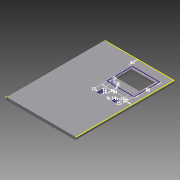
# Autodesk Inventor part: capac frontal
Saved by Autodesk Inventor 2015 SP1 (Build 190203100, 203)
## iProperties
Created: 2015-07-29
Part Number: capac frontal
Material: Generic
Document SubType Name: Modeling
Designer: ubik
Density: 1 g/cm^3
Appearance: Default
Author: ubik
Autodesk Inventor part; units mm, degrees
ref_plane "YZ Plane" through (0, 0, 0) normal (1, 0, 0) x (0, 1, 0)
ref_plane "XZ Plane" through (0, 0, 0) normal (0, 1, 0) x (-1, 0, 0)
ref_plane "XY Plane" through (0, 0, 0) normal (0, 0, 1) x (1, 0, 0)
sketch "Sketch1" plane through (0, 0, 0) normal (0, 0, 1) x (1, 0, 0)
  line L0 (0, 0) -> (240, 0)
  line L1 (240, 0) -> (240, 340)
  line L2 (240, 340) -> (0, 340)
  line L3 (0, 340) -> (0, 0)
  dimension "d0" = 240
  dimension "d1" = 340
  constraints: 8 end point, 2 parallel, 1 horizontal, 1 perpendicular
  measures "d0" distance of L2.end L1.end
  measures "d1" distance of L1.end L0.end
extrude "Extrusion1" add sketch "Sketch1" along normal blind 8
sketch "Sketch2" plane through (0, 0, 8) normal (0, 0, 1) x (1, 0, 0)
  line L0 (126, 310) -> (220, 310)
  line L1 (220, 310) -> (220, 222)
  line L2 (220, 222) -> (126, 222)
  line L3 (126, 222) -> (126, 310)
  line L4 (240, 0) -> (240, 340) projected
  line L5 (240, 340) -> (0, 340) projected
  line L6 (141, 187) -> (152, 187)
  line L7 (152, 187) -> (152, 173)
  line L8 (152, 173) -> (141, 173)
  line L9 (141, 173) -> (141, 187)
  line L10 (194, 187) -> (205, 187)
  line L11 (205, 187) -> (205, 173)
  line L12 (205, 173) -> (194, 173)
  line L13 (194, 173) -> (194, 187)
  circle A0 centre (135, 231) radius 4
  point P0 (0, 0)
  dimension "d4" = 94
  dimension "d5" = 88
  dimension "d6" = 20
  dimension "d7" = 30
  dimension "d8" = 9
  dimension "d9" = 9
  dimension "d10" = 8
  dimension "d11" = 11
  dimension "d12" = 14
  dimension "d13" = 11
  dimension "d14" = 14
  dimension "d15" = 15
  dimension "d16" = 15
  dimension "d17" = 35
  constraints: 24 end point, 6 parallel, 3 horizontal, 3 perpendicular, 1 centre point, 1 point on line
  measures "d4" distance of L1.end L2.end
  measures "d5" distance of L0.end L1.end
  measures "d6" distance between parallel lines of L4 L1
  measures "d7" distance between parallel lines of L5 L0
  measures "d8" distance from line of L2 A0.centre
  measures "d9" distance from line of L3 A0.centre
  measures "d10" diameter of A0
  measures "d11" distance of L6.start L6.end
  measures "d12" distance of L6.end L7.end
  measures "d13" distance of L10.start L10.end
  measures "d14" distance of L12.end L10.start
  measures "d15" distance between parallel lines of L3 L9
  measures "d16" distance between parallel lines of L1 L11
  measures "d17" distance between parallel lines of L2 L6
extrude "Extrusion2" cut sketch "Sketch2" against normal through all contours L6 L7 L8 L9 | L10 L11 L12 L13 | A0
sketch "Sketch3" plane through (0, 0, 0) normal (0, 0, -1) x (-1, 0, 0)
  line L0 (-220, 310) -> (-126, 310)
  line L1 (-126, 310) -> (-126, 222)
  line L2 (-126, 222) -> (-220, 222)
  line L3 (-220, 222) -> (-220, 310)
  line L4 (-240, 340) -> (0, 340) projected
  line L5 (-240, 0) -> (-240, 340) projected
  point P0 (0, 0)
  dimension "d20" = 94
  dimension "d21" = 30
  dimension "d22" = 88
  dimension "d23" = 20
  constraints: 8 end point, 2 parallel, 1 horizontal, 1 perpendicular
  measures "d20" distance of L0.start L0.end
  measures "d21" distance between parallel lines of L4 L0
  measures "d22" distance of L2.end L0.start
  measures "d23" distance between parallel lines of L5 L3
extrude "Extrusion3" cut sketch "Sketch3" against normal blind 3.5
sketch "Sketch4" plane through (0, 0, 3.5) normal (0, 0, -1) x (-1, 0, 0)
  line L0 (-212, 300) -> (-133, 300)
  line L1 (-133, 300) -> (-133, 249)
  line L2 (-133, 249) -> (-212, 249)
  line L3 (-212, 249) -> (-212, 300)
  line L4 (-220, 222) -> (-220, 310) projected
  line L5 (-126, 310) -> (-126, 222) projected
  line L6 (-220, 310) -> (-126, 310) projected
  line L7 (-126, 222) -> (-220, 222) projected
  point P0 (0, 0)
  dimension "d26" = 8
  dimension "d27" = 7
  dimension "d28" = 10
  dimension "d29" = 27
  constraints: 8 end point, 2 parallel, 1 horizontal, 1 perpendicular
  measures "d26" distance between parallel lines of L4 L3
  measures "d27" distance between parallel lines of L5 L1
  measures "d28" distance between parallel lines of L6 L0
  measures "d29" distance between parallel lines of L7 L2
extrude "Extrusion4" cut sketch "Sketch4" against normal through all contours L0 L1 L2 L3
equation "\"d13\" = d11"
equation "\"d14\" = d12"
body "Solid1"
